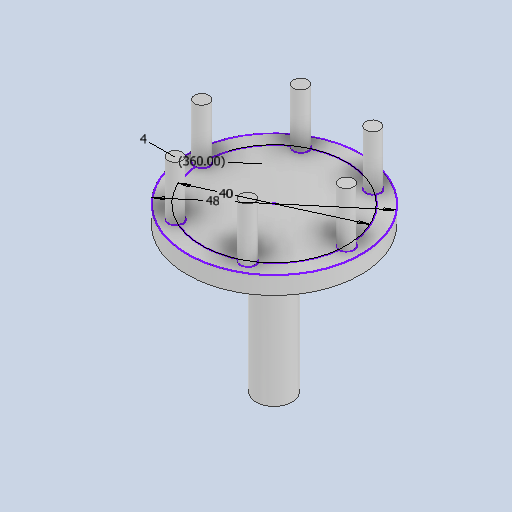
# Autodesk Inventor part: Output_shaft
Saved by Autodesk Inventor 2022 (Build 260153000, 153)
## iProperties
Created: 2021-07-18
Part Number: Output_shaft
Material: Generic
Document SubType Name: Modeling
Designer: Madhav
Density: 1 g/cm^3
Appearance: Default
Author: Madhav
Autodesk Inventor part; units mm, degrees
ref_plane "YZ Plane" through (0, 0, 0) normal (1, 0, 0) x (0, 1, 0)
ref_plane "XZ Plane" through (0, 0, 0) normal (0, 1, 0) x (-1, 0, 0)
ref_plane "XY Plane" through (0, 0, 0) normal (0, 0, 1) x (1, 0, 0)
sketch "Sketch1" plane through (0, 0, 0) normal (0, 1, 0) x (-1, 0, 0)
  circle A0 centre (0, 0) radius 20
  circle A1 centre (20, 0) radius 2
  circle A2 centre (10, 17.3205) radius 2
  circle A3 centre (-10, 17.3205) radius 2
  circle A4 centre (-20, 0) radius 2
  circle A5 centre (-10, -17.3205) radius 2
  circle A6 centre (10, -17.3205) radius 2
  circle A7 centre (0, 0) radius 24
  dimension "d16" = 40
  dimension "d17" = 4
  dimension "d20" = 360
  dimension "d22" = 48
  constraints: 7 centre point, 2 coincident, 1 horizontal alignment, 15 other
  measures "d17" diameter of A1
  measures "d22" diameter of A7
extrude "Extrusion1" add sketch "Sketch1" against normal blind 5 contours A0 A1 | A0 A1 | A1 A0 A6 A5 A4 A3 A2 | A2 A0 | A0 A2 | A6 A0 | A0 A6 | A3 A0 | A0 A3 | A5 A0 | A0 A5 | A4 A0 | A0 A4 | A7
sketch "Sketch2" plane through (0, -5, 0) normal (0, -1, 0) x (1, 0, 0)
  circle A0 centre (0, 0) radius 5
  dimension "d13" = 10
  constraints: 1 centre point, 1 coincident
  measures "d13" diameter of A0
extrude "Extrusion3" add sketch "Sketch2" along normal blind 40
extrude "Extrusion4" add sketch "Sketch1" along normal blind 15 contours A0 A1 | A0 A1 | A2 A0 | A0 A2 | A6 A0 | A0 A6 | A3 A0 | A0 A3 | A5 A0 | A0 A5 | A4 A0 | A0 A4
body "Solid1"
